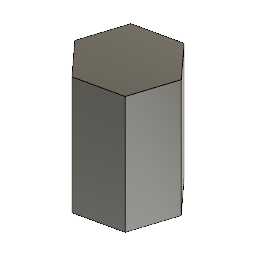
Polygon Wedge Print (Autodesk Fusion 360 design; units mm, degrees)
Autodesk Fusion 360 part; units mm, degrees
sketch "Sketch1" plane through (0, 0, 0) normal (0, 0, 1) x (1, 0, 0)
  line L0 (2.5647, -2.804) -> (3.7107, 0.819)
  line L1 (3.7107, 0.819) -> (1.146, 3.6231)
  line L2 (1.146, 3.6231) -> (-2.5647, 2.804)
  line L3 (-2.5647, 2.804) -> (-3.7107, -0.819)
  line L4 (-3.7107, -0.819) -> (-1.146, -3.6231)
  line L5 (-1.146, -3.6231) -> (2.5647, -2.804)
  dimension "d1" = 3.8
  measures "d1" distance of L0.start origin
extrude "Extrude1" add sketch "Sketch1" along normal blind 10
